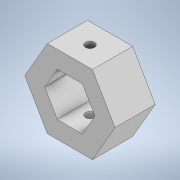
# Autodesk Inventor part: Hombro_Ejes
Saved by Autodesk Inventor 2022 (Build 260153000, 153)
## iProperties
Created: 2022-02-21
Part Number: Hombro_Ejes
Material: Generic
Document SubType Name: Modeling
Designer: katha
Density: 1 g/cm^3
Appearance: Default
Author: katha
Autodesk Inventor part; units mm, degrees
ref_plane "YZ Plane" through (0, 0, 0) normal (1, 0, 0) x (0, 1, 0)
ref_plane "XZ Plane" through (0, 0, 0) normal (0, 1, 0) x (-1, 0, 0)
ref_plane "XY Plane" through (0, 0, 0) normal (0, 0, 1) x (1, 0, 0)
sketch "Sketch5" plane through (0, 0, 0) normal (0, 0, 1) x (1, 0, 0)
  line L0 (0, 0) -> (3.1, 0) construction
  circle A0 centre (0, 0) radius 3.1 construction
  line L1 (0, 0) -> (1.55, 2.6847) construction
  line L2 (0, 0) -> (-1.55, 2.6847) construction
  line L3 (0, 0) -> (-3.1, 0) construction
  line L4 (0, 0) -> (-1.55, -2.6847) construction
  line L5 (0, 0) -> (1.55, -2.6847) construction
  line L6 (-1.55, 2.6847) -> (1.55, 2.6847) construction
  line L7 (1.55, 2.6847) -> (3.1, 0) construction
  line L8 (3.1, 0) -> (1.55, -2.6847) construction
  line L9 (-1.55, 2.6847) -> (-3.1, 0) construction
  line L10 (-3.1, 0) -> (-1.55, -2.6847) construction
  line L11 (-1.55, -2.6847) -> (1.55, -2.6847) construction
  line L12 (3.6196, 0) -> (1.8098, 3.1347)
  line L13 (1.8098, 3.1347) -> (-1.8098, 3.1347)
  line L14 (-1.8098, 3.1347) -> (-3.6196, 0)
  line L15 (-3.6196, 0) -> (-1.8098, -3.1347)
  line L16 (-1.8098, -3.1347) -> (1.8098, -3.1347)
  line L17 (1.8098, -3.1347) -> (3.6196, 0)
  line L18 (3.2532, 5.6347) -> (6.5064, 0)
  line L19 (6.5064, 0) -> (3.2532, -5.6347)
  line L20 (3.2532, -5.6347) -> (-3.2532, -5.6347)
  line L21 (-3.2532, -5.6347) -> (-6.5064, 0)
  line L22 (-6.5064, 0) -> (-3.2532, 5.6347)
  line L23 (-3.2532, 5.6347) -> (3.2532, 5.6347)
  dimension "d9" = 3.1
  dimension "d12" = 360
  dimension "d14" = 0.45
  dimension "d15" = 2.5
  constraints: 48 end point, 3 horizontal, 1 coincident, 1 horizontal alignment, 31 other
  measures "d9" distance of L0.start L0.end
  measures "d14" distance between parallel lines of L7 L12
  measures "d15" distance between parallel lines of L12 L18
extrude "Extrusion4" add sketch "Sketch5" along normal blind 5.8
sketch "Sketch6" plane through (-3.2532, 5.6347, 0) normal (0, 1, 0) x (1, 0, 0)
  line L0 (0, -5.8) -> (6.5064, -5.8) projected
  line L1 (3.2532, -5.8) -> (3.2532, 0) construction
  line L2 (0, 0) -> (0, -5.8) projected
  line L3 (0, -2.9) -> (6.5064, -2.9) construction
  line L4 (6.5064, 0) -> (6.5064, -5.8) projected
  circle A0 centre (3.2532, -2.9) radius 0.65
  dimension "d18" = 1.3
  constraints: 4 end point, 4 midpoint, 1 centre point, 1 vertical
  measures "d18" diameter of A0
extrude "Extrusion5" cut sketch "Sketch6" against normal blind 15
body "Solid2"
